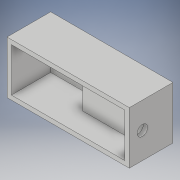
# Autodesk Inventor part: escbox
Saved by Autodesk Inventor 2017 (Build 210142000, 142)
## iProperties
Created: 2017-08-13
Part Number: escbox
Material: Generic
Document SubType Name: Modeling
Designer: Kai
Density: 1 g/cm^3
Appearance: Default
Author: Kai
Autodesk Inventor part; units mm, degrees
ref_plane "YZ Plane" through (0, 0, 0) normal (1, 0, 0) x (0, 1, 0)
ref_plane "XZ Plane" through (0, 0, 0) normal (0, 1, 0) x (-1, 0, 0)
ref_plane "XY Plane" through (0, 0, 0) normal (0, 0, 1) x (1, 0, 0)
sketch "Sketch1" plane through (0, 0, 0) normal (0, 0, 1) x (1, 0, 0)
  line L0 (0, 0) -> (-88.9, 0)
  line L1 (-88.9, 0) -> (-88.9, 38.1)
  line L2 (-88.9, 38.1) -> (0, 38.1)
  line L3 (0, 38.1) -> (0, 0)
  circle A0 centre (-69.85, 19.05) radius 10.5029
  dimension "d0" = 88.9
  dimension "d1" = 38.1
  dimension "d2" = 21.0058
  dimension "d3" = 19.05
  dimension "d4" = 19.05
  constraints: 8 end point, 2 parallel, 1 centre point, 1 horizontal, 1 perpendicular
  measures "d0" distance of L1.end L2.end
  measures "d1" distance of L0.end L1.end
  measures "d2" diameter of A0
  measures "d3" distance from line of L1 A0.centre
  measures "d4" distance from line of L0 A0.centre
extrude "Extrusion1" add sketch "Sketch1" along normal blind 3.175
sketch "Sketch2" plane through (0, 0, 3.175) normal (0, 0, 1) x (1, 0, 0)
  line L0 (-88.9, 38.1) -> (-88.9, 0) projected
  line L1 (0, 0) -> (0, 38.1) projected
  line L2 (-88.9, 38.1) -> (0, 38.1)
  line L3 (0, 38.1) -> (0, 0)
  line L4 (0, 0) -> (-88.9, 0)
  line L5 (-88.9, 0) -> (-88.9, 38.1)
  line L6 (-3.175, 34.925) -> (-85.725, 34.925)
  line L7 (-85.725, 34.925) -> (-85.725, 3.175)
  line L8 (-85.725, 3.175) -> (-3.175, 3.175)
  line L9 (-3.175, 3.175) -> (-3.175, 34.925)
  dimension "d7" = 3.175
  constraints: 16 end point, 4 parallel, 2 perpendicular, 1 horizontal, 3 other
  measures "d7" distance between parallel lines of L2 L6
extrude "Extrusion2" add sketch "Sketch2" along normal blind 28.575
sketch "Sketch3" plane through (0, 0, 3.175) normal (0, 0, 1) x (1, 0, 0)
  line L0 (-3.175, 34.925) -> (-3.175, 3.175) projected
  line L1 (-85.725, 3.175) -> (-3.175, 3.175) projected
  line L2 (-3.175, 34.925) -> (-49.8348, 34.925)
  line L3 (-49.8348, 34.925) -> (-49.8348, 3.175)
  line L4 (-49.8348, 3.175) -> (-3.175, 3.175)
  line L5 (-3.175, 3.175) -> (-3.175, 34.925)
  point P0 (0, 0)
  dimension "d10" = 46.6598
  constraints: 8 end point, 2 parallel, 1 horizontal, 1 perpendicular, 1 point on line
  measures "d10" distance of L4.end L3.end
extrude "Extrusion3" add sketch "Sketch3" along normal blind 12.7
sketch "Sketch4" plane through (0, 0, 0) normal (1, 0, 0) x (0, 0, -1)
  circle A0 centre (-22.225, 19.05) radius 3.81
  line L0 (-31.75, 0) -> (-31.75, 38.1) projected
  point P0 (0, 0)
  dimension "d13" = 7.62
  dimension "d14" = 9.525
  constraints: 1 centre point
  measures "d13" diameter of A0
  measures "d14" distance from line of L0 A0.centre
extrude "Extrusion4" cut sketch "Sketch4" against normal blind 19.05
body "Solid1"
